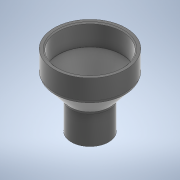
# Autodesk Inventor part: Chute
Saved by Autodesk Inventor 2020.2 (Build 242310000, 310)
## iProperties
Created: 2020-10-16
Part Number: Chute
Material: Generic
Document SubType Name: Modeling
Designer: JK
Density: 1 g/cm^3
Appearance: Smooth - Black
Author: JK
Autodesk Inventor part; units mm, degrees
ref_plane "YZ Plane" through (0, 0, 0) normal (1, 0, 0) x (0, 1, 0)
ref_plane "XZ Plane" through (0, 0, 0) normal (0, 1, 0) x (-1, 0, 0)
ref_plane "XY Plane" through (0, 0, 0) normal (0, 0, 1) x (1, 0, 0)
sketch "Sketch1" plane through (0, 0, 0) normal (0, 1, 0) x (-1, 0, 0)
  circle A0 centre (0, 0) radius 10.3
  circle A1 centre (0, 0) radius 13.3
  dimension "d0" = 20.6
  dimension "d1" = 3
  constraints: 2 centre point, 2 coincident
  measures "d0" diameter of A0
  measures "d1" radial gap between concentric circles of A1 A0
extrude "Extrusion1" add sketch "Sketch1" along normal blind 25
sketch "Sketch2" plane through (0, 0, 0) normal (0, 0, 1) x (1, 0, 0)
  circle A0 centre (0, 4) radius 16
  line L0 (13.3, 25) -> (-13.3, 25) projected
  line L1 (0, 25) -> (0, 20)
  point P0 (0, 0)
  dimension "d4" = 32
  dimension "d5" = 5
  constraints: 2 end point, 2 vertical alignment, 1 midpoint, 1 perpendicular, 2 other
  measures "d5" distance of L1.start L1.end
extrude "Extrusion2" cut sketch "Sketch2" against normal through all both and the other way through all
sketch "Sketch4" plane through (0, 0, 0) normal (1, 0, 0) x (0, 1, 0)
  line L0 (20, 13.3) -> (25, 13.3) projected
  line L1 (25, 13.3) -> (40, 25.6)
  line L2 (40, 25.6) -> (55, 25.6)
  line L3 (55, 25.6) -> (55, 22.6)
  line L4 (55, 22.6) -> (40, 22.6)
  line L5 (25, 10.3) -> (25, -10.3) projected
  line L6 (40, 22.6) -> (25, 10.3)
  line L7 (0, 0) -> (85.2959, 0)
  line L8 (25, 13.3) -> (25, 10.3)
  line L9 (25, -13.3) -> (25, 13.3) projected
  point P0 (25, 0)
  dimension "d8" = 22.6
  dimension "d9" = 3
  dimension "d11" = 15
  dimension "d12" = 30
  constraints: 14 end point, 2 parallel, 2 perpendicular, 1 collinear, 1 horizontal, 1 midpoint, 1 point on line, 1 vertical alignment
  measures "d8" vertical distance of L3.end point (25, 0)
  measures "d9" distance between parallel lines of L4 L2
  measures "d11" horizontal distance of L4.end point (25, 0)
  measures "d12" horizontal distance of point (25, 0) L3.end
revolve "Revolution1" add sketch "Sketch4" angle 360 about axis through (0, 0, 0) along (0, 1, 0)
chamfer "Chamfer1" distance 1 angle 45 5 edges at (0, 40, -25.6) (0, 55, -22.6) (10.3, 16.2438, -0.0012) (9.4045, 25, -9.4045) (-9.4045, 25, 9.4045)
sketch "Sketch5" plane through (0, 0, 0) normal (0, 1, 0) x (-1, 0, 0)
  circle A0 centre (0, 0) radius 13.9341 projected
  circle A1 centre (0, 0) radius 35.7982
  point P0 (0, 0)
  constraints: 1 centre point, 1 coincident
extrude "Extrusion3" cut sketch "Sketch5" along normal blind 24 contours A0 | A1
sketch "Sketch6" plane through (0, 24, 0) normal (0, -1, 0) x (1, 0, 0)
  circle A0 centre (0, 0) radius 10.3
  circle A1 centre (0, 0) radius 13.3
  constraints: 2 centre point, 2 coincident
extrude "Extrusion4" add sketch "Sketch6" along normal blind 20
sketch "Sketch7" plane through (0, 4, 0) normal (0, -1, 0) x (1, 0, 0)
  circle A0 centre (0, 0) radius 6.75
  circle A1 centre (0, 0) radius 13.3 projected
  circle A2 centre (0, 0) radius 10.3 projected
  dimension "d21" = 13.5
  constraints: 1 centre point, 1 coincident
  measures "d21" diameter of A0
extrude "Extrusion5" add sketch "Sketch7" against normal blind 21 contours A1 | A2
chamfer "Chamfer2" distance 10 angle 15 1 edges at (-6.75, 25, 0) measured on face at (-6.75, 24.5, 0)
fillet "Fillet1" radius 2 1 edges at (-6.75, 4, 0)
sketch "Sketch8" plane through (0, 55, 0) normal (0, 1, 0) x (1, 0, 0)
  circle A0 centre (0, 0) radius 22.8
  dimension "d28" = 45.6
  constraints: 1 centre point, 1 coincident
  measures "d28" diameter of A0
extrude "Extrusion6" cut sketch "Sketch8" against normal blind 15
body "Solid1"
